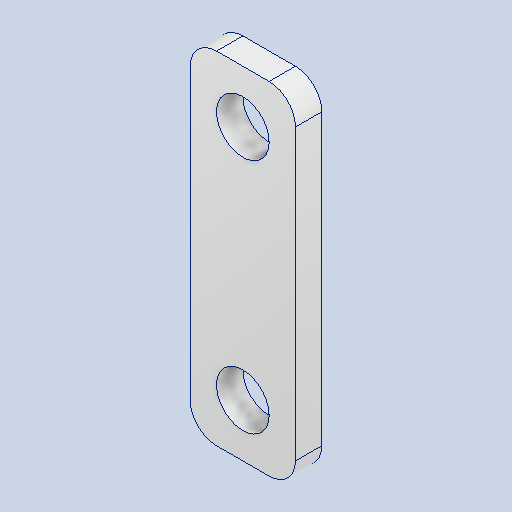
# Autodesk Inventor part: Servo arm
Saved by Autodesk Inventor 2023 (Build 270158000, 158)
## iProperties
Created: 2022-06-23
Part Number: Servo arm
Material: Aluminum 6061
Document SubType Name: Modeling
Designer: earls
Density: 2.7 g/cm^3
Appearance: Aluminum - Flat
Author: earls
Autodesk Inventor part; units mm, degrees
ref_plane "YZ Plane" through (0, 0, 0) normal (1, 0, 0) x (0, 1, 0)
ref_plane "XZ Plane" through (0, 0, 0) normal (0, 1, 0) x (-1, 0, 0)
ref_plane "XY Plane" through (0, 0, 0) normal (0, 0, 1) x (1, 0, 0)
sketch "Sketch1" plane through (0, 0, 0) normal (0, 0, 1) x (1, 0, 0)
  line L0 (-5, 0) -> (-15, 0)
  line L1 (-20, 5) -> (-20, 60)
  line L2 (-15, 65) -> (-5, 65)
  line L3 (0, 60) -> (0, 5)
  circle A0 centre (-10, 55) radius 5
  circle A1 centre (-10, 10) radius 5
  arc A2 (-15, 65) -> (-20, 60) centre (-15, 60) ccw
  arc A3 (0, 60) -> (-5, 65) centre (-5, 60) ccw
  arc A4 (-20, 5) -> (-15, 0) centre (-15, 5) ccw
  arc A5 (-5, 0) -> (0, 5) centre (-5, 5) ccw
  point P0 (0, 0)
  point P1 (-20, 65)
  point P2 (-20, 0)
  point P3 (0, 65)
  dimension "d0" = 20
  dimension "d1" = 65
  dimension "d2" = 10
  dimension "d3" = 45
  dimension "d4" = 10
  dimension "d5" = 5
  constraints: 8 end point, 8 point on circle, 8 point on line, 8 tangent, 6 centre point, 4 equal radius, 2 parallel, 1 horizontal, 1 perpendicular
  measures "d0" distance of point (-20, 65) point (0, 65)
  measures "d1" distance of point (-20, 0) point (-20, 65)
  measures "d2" diameter of A0
  measures "d3" distance of A1.centre A0.centre
  measures "d4" distance from line of A0.centre L2
  measures "d5" radius of A2
extrude "Extrusion1" add sketch "Sketch1" along normal mid plane 5
sketch "Sketch2" plane through (0, 0, 2.5) normal (0, 0, 1) x (1, 0, 0)
  line L0 (-5, 65) -> (-15, 65) projected
  arc A0 (-15, 65) -> (-20, 60) centre (-15, 60) ccw projected
  line L1 (-20, 60) -> (-20, 5) projected
  arc A1 (-20, 5) -> (-15, 0) centre (-15, 5) ccw projected
  line L2 (-15, 0) -> (-5, 0) projected
  arc A2 (-5, 0) -> (0, 5) centre (-5, 5) ccw projected
  line L3 (0, 5) -> (0, 60) projected
  arc A3 (0, 60) -> (-5, 65) centre (-5, 60) ccw projected
  circle A4 centre (-10, 10) radius 5 projected
  circle A5 centre (-10, 55) radius 5 projected
  point P0 (0, 0)
body "Solid1"
